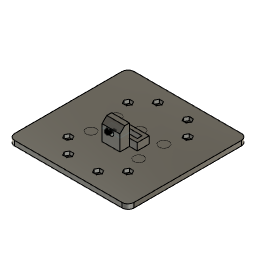
SidePanel-Back (Autodesk Fusion 360 design; units mm, degrees)
Autodesk Fusion 360 part; units mm, degrees
note: some values were not read from the file. Set by a fixed rule: which sketch regions a step uses.
sketch "Skizze1" plane through (0, 0, 0) normal (0, 0, 1) x (1, 0, 0)
  line L0 (0, 0) -> (100, 0)
  line L1 (100, 0) -> (100, 100)
  line L2 (100, 100) -> (0, 100)
  line L3 (0, 100) -> (0, 0)
  circle A0 centre (5, 95) radius 5
  circle A1 centre (5, 5) radius 5
  circle A2 centre (95, 5) radius 5
  circle A3 centre (95, 95) radius 5
  line L4 (39, 46.75) -> (61, 46.75)
  line L5 (61, 46.75) -> (61, 50.75)
  line L6 (61, 50.75) -> (39, 50.75)
  line L7 (39, 50.75) -> (39, 46.75)
  line L8 (39, 48.75) -> (61, 48.75)
  line L9 (50, 50.75) -> (50, 46.75)
  dimension "d1" = 100
  dimension "d2" = 100
  dimension "d5" = 22
  dimension "d6" = 4
  dimension "d7" = 50
  dimension "d8" = 48.75
  constraint horizontal L0
  constraint vertical L1
  constraint horizontal L2
  constraint vertical L3
  constraint coincident L0.start L3.end
  constraint tangent L2 A0
  constraint tangent L0 A1
  constraint tangent L1 A2
  constraint tangent L2 A3
  constraint horizontal L4
  constraint vertical L5
  constraint horizontal L6
  constraint vertical L7
  constraint midpoint L7 L8.start
  constraint midpoint L5 L8.end
  constraint midpoint L6 L9.start
  constraint midpoint L4 L9.end
  measures "d1" distance of L0.start L0.end
  measures "d2" distance of L0.start L2.end
  measures "d5" distance of L4.start L4.end
  measures "d6" distance of L4.start L6.end
  measures "d7" distance of L3 L9
  measures "d8" distance of L0 L8
extrude "Extrusion1" add sketch "Skizze1" along normal blind 4 contours L0 L1 L2 L3 A0 A1 A2 A3 | A1 | A2 | A0 | A3
sketch "Skizze2" plane through (0, 0, 4) normal (0, 0, 1) x (-1, 0, 0)
  line L0 (-39, -46.75) -> (-39, -50.75)
  line L1 (-39, -50.75) -> (-61, -50.75)
  line L2 (-61, -50.75) -> (-61, -46.75)
  line L3 (-61, -46.75) -> (-39, -46.75)
  arc A0 (-100, -95) -> (-95, -100) centre (-95, -95) ccw
  line L4 (-95, -100) -> (-5, -100)
  arc A1 (-5, -100) -> (0, -95) centre (-5, -95) ccw
  line L5 (0, -95) -> (0, -5)
  arc A2 (0, -5) -> (-5, 0) centre (-5, -5) ccw
  line L6 (-5, 0) -> (-95, 0)
  arc A3 (-95, 0) -> (-100, -5) centre (-95, -5) ccw
  line L7 (-100, -5) -> (-100, -95)
  line L8 (-39, -53.75) -> (-64, -53.75)
  line L9 (-64, -53.75) -> (-64, -43.75)
  line L10 (-64, -43.75) -> (-39, -43.75)
  line L11 (-39, -43.75) -> (-39, -53.75)
  line L12 (-39, -48.75) -> (-42, -48.75)
  arc A4 (-39, -53.75) -> (-39, -43.75) centre (-39, -48.75) ccw
  dimension "d9" = 3
  dimension "d10" = 3
  dimension "d11" = 3
  constraint horizontal L8
  constraint vertical L9
  constraint horizontal L10
  constraint vertical L11
  constraint collinear L0 L11
  constraint midpoint L11 L12.start
  constraint perpendicular L11 L12
  constraint coincident L12.start A4.centre
  measures "d9" distance of L1 L8
  measures "d10" distance of L3 L10
  measures "d11" distance of L2 L9
extrude "Extrusion2" add sketch "Skizze2" along normal blind 6 contours L0 L11 A4 | L1 L2 L3 L8 L9 L10 L11
sketch "Skizze3" plane through (0, 0, 0) normal (0, 0, -1) x (1, 0, 0)
  line L0 (39, -50.75) -> (39, -46.75)
  line L1 (39, -46.75) -> (61, -46.75)
  line L2 (61, -46.75) -> (61, -50.75)
  line L3 (61, -50.75) -> (39, -50.75)
  arc A0 (95, -100) -> (100, -95) centre (95, -95) ccw
  line L4 (100, -95) -> (100, -5)
  arc A1 (100, -5) -> (95, 0) centre (95, -5) ccw
  line L5 (95, 0) -> (5, 0)
  arc A2 (5, 0) -> (0, -5) centre (5, -5) ccw
  line L6 (0, -5) -> (0, -95)
  arc A3 (0, -95) -> (5, -100) centre (5, -95) ccw
  line L7 (5, -100) -> (95, -100)
  line L8 (23, -36) -> (3, -36)
  line L9 (3, -36) -> (3, -5)
  line L10 (3, -5) -> (23, -5)
  line L11 (23, -5) -> (23, -36)
  line L12 (23, -36) -> (18, -36)
  line L13 (18, -36) -> (18, -21)
  line L14 (18, -21) -> (23, -21)
  line L15 (23, -21) -> (23, -36)
  dimension "d15" = 20
  dimension "d16" = 31
  dimension "d17" = 5
  dimension "d18" = 3
  dimension "d62" = 5
  dimension "d63" = 15
  constraint horizontal L8
  constraint vertical L9
  constraint horizontal L10
  constraint vertical L11
  constraint horizontal L12
  constraint vertical L13
  constraint horizontal L14
  constraint vertical L15
  measures "d15" distance of L8.start L8.end
  measures "d16" distance of L8.start L10.end
  measures "d17" distance of L5 L10
  measures "d18" distance of L6 L9
  measures "d62" distance of L13.end L14.end
  measures "d63" distance of L12.end L13.end
extrude "Extrusion3" cut sketch "Skizze3" against normal blind 2 contours L8 L9 L10 L11 L13 L14
sketch "Skizze4" plane through (0, 0, 0) normal (0, 0, -1) x (1, 0, 0)
  line L0 (3, -36) -> (3, -5)
  line L1 (3, -5) -> (23, -5)
  line L2 (23, -5) -> (23, -21)
  line L3 (18, -36) -> (3, -36)
  line L4 (39, -50.75) -> (39, -46.75)
  line L5 (39, -46.75) -> (61, -46.75)
  line L6 (61, -46.75) -> (61, -50.75)
  line L7 (61, -50.75) -> (39, -50.75)
  arc A0 (95, -100) -> (100, -95) centre (95, -95) ccw
  line L8 (100, -95) -> (100, -5)
  arc A1 (100, -5) -> (95, 0) centre (95, -5) ccw
  line L9 (95, 0) -> (5, 0)
  arc A2 (5, 0) -> (0, -5) centre (5, -5) ccw
  line L10 (0, -5) -> (0, -95)
  arc A3 (0, -95) -> (5, -100) centre (5, -95) ccw
  line L11 (5, -100) -> (95, -100)
  line L12 (25, -25) -> (75, -25)
  line L13 (75, -25) -> (75, -75)
  line L14 (75, -75) -> (25, -75)
  line L15 (25, -75) -> (25, -25)
  circle A4 centre (25, -25) radius 1.75
  circle A5 centre (75, -25) radius 1.75
  circle A6 centre (75, -75) radius 1.75
  circle A7 centre (25, -75) radius 1.75
  line L16 (37.5, -12.5) -> (62.5, -12.5)
  line L17 (62.5, -12.5) -> (62.5, -87.5)
  line L18 (62.5, -87.5) -> (37.5, -87.5)
  line L19 (37.5, -87.5) -> (37.5, -12.5)
  circle A8 centre (37.5, -12.5) radius 1.75
  circle A9 centre (62.5, -12.5) radius 1.75
  circle A10 centre (62.5, -87.5) radius 1.75
  circle A11 centre (37.5, -87.5) radius 1.75
  line L20 (23, -21) -> (18, -21)
  line L21 (18, -21) -> (18, -36)
  dimension "d21" = 50
  dimension "d22" = 50
  dimension "d23" = 25
  dimension "d24" = 25
  dimension "d25" = 3.5
  dimension "d26" = 3.5
  dimension "d27" = 3.5
  dimension "d28" = 3.5
  dimension "d29" = 25
  dimension "d30" = 75
  dimension "d31" = 12.5
  dimension "d32" = 37.5
  dimension "d33" = 3.5
  dimension "d34" = 3.5
  dimension "d35" = 3.5
  dimension "d36" = 3.5
  constraint horizontal L12
  constraint vertical L13
  constraint horizontal L14
  constraint vertical L15
  constraint coincident L12.start L15.end
  constraint coincident L12.end L13.start
  constraint coincident L13.end L14.start
  constraint coincident L14.end L15.start
  constraint horizontal L16
  constraint vertical L17
  constraint horizontal L18
  constraint vertical L19
  constraint coincident L16.start L19.end
  constraint coincident L16.end L17.start
  constraint coincident L17.end L18.start
  constraint coincident L18.end L19.start
  measures "d21" distance of L12.start L12.end
  measures "d22" distance of L12.end L13.end
  measures "d23" distance of L8 L13
  measures "d24" distance of L11 L14
  measures "d25" diameter of A4
  measures "d26" diameter of A5
  measures "d27" diameter of A6
  measures "d28" diameter of A7
  measures "d29" distance of L16.start L16.end
  measures "d30" distance of L16.start L18.end
  measures "d31" distance of L9 L16
  measures "d32" distance of L8 L17
  measures "d33" diameter of A8
  measures "d34" diameter of A9
  measures "d35" diameter of A10
  measures "d36" diameter of A11
extrude "Extrusion4" cut sketch "Skizze4" against normal blind 4 contours L12 L15 A4 | L12 L15 A4 | L14 L15 A7 | L14 L15 A7 | L16 L19 A8 | L16 L19 A8 | L12 L13 A5 | L12 L13 A5 | L16 L17 A9 | L16 L17 A9 | L18 L19 A11 | L18 L19 A11 | L13 L14 A6 | L13 L14 A6 | L17 L18 A10 | L17 L18 A10
sketch "Skizze5" plane through (0, 0, 4) normal (0, 0, 1) x (-1, 0, 0)
  circle A0 centre (-37.5, -87.5) radius 1.75
  circle A1 centre (-25, -75) radius 1.75
  line L0 (-64, -53.75) -> (-64, -43.75)
  line L1 (-64, -43.75) -> (-39, -43.75)
  arc A2 (-39, -53.75) -> (-39, -43.75) centre (-39, -48.75) ccw
  line L2 (-39, -53.75) -> (-64, -53.75)
  arc A3 (-100, -95) -> (-95, -100) centre (-95, -95) ccw
  line L3 (-95, -100) -> (-5, -100)
  arc A4 (-5, -100) -> (0, -95) centre (-5, -95) ccw
  line L4 (0, -95) -> (0, -5)
  arc A5 (0, -5) -> (-5, 0) centre (-5, -5) ccw
  line L5 (-5, 0) -> (-95, 0)
  arc A6 (-95, 0) -> (-100, -5) centre (-95, -5) ccw
  line L6 (-100, -5) -> (-100, -95)
  line L7 (-34, -90.45) -> (-42, -90.45)
  line L8 (-34, -84.55) -> (-43, -84.55)
  line L9 (-20.1646, -77.9663) -> (-28.1646, -77.9393)
  line L10 (-20.1651, -72.05) -> (-29.1651, -72.05)
  line L11 (0, -50) -> (-100, -50)
  line L12 (-50, -100) -> (-50, 0)
  circle A7 centre (-50, -50) radius 3
  line L13 (-36.6952, -82.9939) -> (-32.6952, -89.9221)
  line L14 (-41.8048, -85.9439) -> (-37.3048, -93.7381)
  line L15 (-41.8048, -89.0561) -> (-37.8048, -82.1279)
  line L16 (-36.6952, -92.0061) -> (-32.1952, -84.2119)
  line L17 (-24.8488, -69.3292) -> (-20.8722, -76.2709)
  line L18 (-29.9722, -72.2879) -> (-25.4722, -80.0821)
  line L19 (-29.9866, -77.7044) -> (-25.9633, -70.7897)
  line L20 (-24.8627, -80.6621) -> (-20.3627, -72.8679)
  line L21 (-79.9722, -72.2879) -> (-75.4722, -80.0821)
  line L22 (-70.1646, -77.9663) -> (-78.1646, -77.9393)
  line L23 (-74.8627, -80.6621) -> (-70.3627, -72.8679)
  line L24 (-74.8488, -69.3292) -> (-70.8722, -76.2709)
  line L25 (-70.1651, -72.05) -> (-79.1651, -72.05)
  line L26 (-79.9866, -77.7044) -> (-75.9633, -70.7897)
  line L27 (-29.9722, -22.2879) -> (-25.4722, -30.0821)
  line L28 (-20.1646, -27.9663) -> (-28.1646, -27.9393)
  line L29 (-24.8627, -30.6621) -> (-20.3627, -22.8679)
  line L30 (-24.8488, -19.3292) -> (-20.8722, -26.2709)
  line L31 (-20.1651, -22.05) -> (-29.1651, -22.05)
  line L32 (-29.9866, -27.7044) -> (-25.9633, -20.7897)
  line L33 (-79.9722, -22.2879) -> (-75.4722, -30.0821)
  line L34 (-70.1646, -27.9663) -> (-78.1646, -27.9393)
  line L35 (-74.8627, -30.6621) -> (-70.3627, -22.8679)
  line L36 (-74.8488, -19.3292) -> (-70.8722, -26.2709)
  line L37 (-70.1651, -22.05) -> (-79.1651, -22.05)
  line L38 (-79.9866, -27.7044) -> (-75.9633, -20.7897)
  line L39 (-59, -84.55) -> (-68, -84.55)
  line L40 (-61.6952, -82.9939) -> (-57.6952, -89.9221)
  line L41 (-61.6952, -92.0061) -> (-57.1952, -84.2119)
  line L42 (-59, -90.45) -> (-67, -90.45)
  line L43 (-66.8048, -85.9439) -> (-62.3048, -93.7381)
  line L44 (-66.8048, -89.0561) -> (-62.8048, -82.1279)
  line L45 (-34, -9.55) -> (-43, -9.55)
  line L46 (-36.6952, -7.9939) -> (-32.6952, -14.9221)
  line L47 (-36.6952, -17.0061) -> (-32.1952, -9.2119)
  line L48 (-34, -15.45) -> (-42, -15.45)
  line L49 (-41.8048, -10.9439) -> (-37.3048, -18.7381)
  line L50 (-41.8048, -14.0561) -> (-37.8048, -7.1279)
  line L51 (-59, -9.55) -> (-68, -9.55)
  line L52 (-61.6952, -7.9939) -> (-57.6952, -14.9221)
  line L53 (-61.6952, -17.0061) -> (-57.1952, -9.2119)
  line L54 (-59, -15.45) -> (-67, -15.45)
  line L55 (-66.8048, -10.9439) -> (-62.3048, -18.7381)
  line L56 (-66.8048, -14.0561) -> (-62.8048, -7.1279)
  dimension "d40" = 2.95
  dimension "d41" = 2.95
  dimension "d42" = 2.95
  dimension "d43" = 2.95
  dimension "d78" = 360
  dimension "d80" = 360
  dimension "d83" = -50
  dimension "d84" = 50
  dimension "d87" = -25
  dimension "d88" = 75
  constraint parallel L3 L7
  constraint horizontal L8
  constraint horizontal L10
  constraint midpoint L4 L11.start
  constraint midpoint L6 L11.end
  constraint midpoint L3 L12.start
  constraint midpoint L5 L12.end
  constraint midpoint L11 A7.centre
  measures "d40" distance of A0.centre L7
  measures "d41" distance of A0.centre L8
  measures "d42" distance of A1.centre L9
  measures "d43" distance of A1.centre L10
extrude "Extrusion5" cut sketch "Skizze5" against normal blind 3 contours A0 | L7 L8 L13 L14 L15 L16 | L9 L10 L17 L18 L19 L20 | L21 L22 L23 L24 L25 L26 | L27 L28 L29 L30 L31 L32 | L33 L34 L35 L36 L37 L38 | L39 L40 L41 L42 L43 L44 | L45 L46 L47 L48 L49 L50 | L51 L52 L53 L54 L55 L56
sketch "Skizze6" plane through (0, 0, 4) normal (0, 0, 1) x (-1, 0, 0)
  line L0 (-26.6966, -72.05) -> (-23.2902, -72.05)
  line L1 (-23.3001, -77.9557) -> (-26.7065, -77.9443)
  line L2 (-39.2032, -84.55) -> (-35.7968, -84.55)
  line L3 (-35.7968, -90.45) -> (-39.2032, -90.45)
  line L4 (-64, -53.75) -> (-64, -43.75)
  line L5 (-64, -43.75) -> (-39, -43.75)
  arc A0 (-39, -53.75) -> (-39, -43.75) centre (-39, -48.75) ccw
  line L6 (-39, -53.75) -> (-64, -53.75)
  arc A1 (-100, -95) -> (-95, -100) centre (-95, -95) ccw
  line L7 (-95, -100) -> (-5, -100)
  arc A2 (-5, -100) -> (0, -95) centre (-5, -95) ccw
  line L8 (0, -95) -> (0, -5)
  arc A3 (0, -5) -> (-5, 0) centre (-5, -5) ccw
  line L9 (-5, 0) -> (-95, 0)
  arc A4 (-95, 0) -> (-100, -5) centre (-95, -5) ccw
  line L10 (-100, -5) -> (-100, -95)
  line L11 (-42.5, -43.75) -> (-57.5, -43.75)
  line L12 (-57.5, -43.75) -> (-57.5, -35.75)
  line L13 (-57.5, -35.75) -> (-42.5, -35.75)
  line L14 (-42.5, -35.75) -> (-42.5, -43.75)
  line L15 (-28.4097, -74.9943) -> (-26.6966, -72.05)
  line L16 (-23.2902, -72.05) -> (-21.5969, -75.0057)
  line L17 (-21.5969, -75.0057) -> (-23.3001, -77.9557)
  line L18 (-26.7065, -77.9443) -> (-28.4097, -74.9943)
  line L19 (-40.9064, -87.5) -> (-39.2032, -84.55)
  line L20 (-35.7968, -84.55) -> (-34.0936, -87.5)
  line L21 (-34.0936, -87.5) -> (-35.7968, -90.45)
  line L22 (-39.2032, -90.45) -> (-40.9064, -87.5)
  line L23 (-28.4097, -24.9943) -> (-26.6966, -22.05)
  line L24 (-26.6966, -22.05) -> (-23.2902, -22.05)
  line L25 (-23.2902, -22.05) -> (-21.5969, -25.0057)
  line L26 (-21.5969, -25.0057) -> (-23.3001, -27.9557)
  line L27 (-23.3001, -27.9557) -> (-26.7065, -27.9443)
  line L28 (-26.7065, -27.9443) -> (-28.4097, -24.9943)
  line L29 (-65.9064, -87.5) -> (-64.2032, -84.55)
  line L30 (-64.2032, -84.55) -> (-60.7968, -84.55)
  line L31 (-60.7968, -84.55) -> (-59.0936, -87.5)
  line L32 (-59.0936, -87.5) -> (-60.7968, -90.45)
  line L33 (-60.7968, -90.45) -> (-64.2032, -90.45)
  line L34 (-64.2032, -90.45) -> (-65.9064, -87.5)
  line L35 (-40.9064, -12.5) -> (-39.2032, -9.55)
  line L36 (-39.2032, -9.55) -> (-35.7968, -9.55)
  line L37 (-35.7968, -9.55) -> (-34.0936, -12.5)
  line L38 (-34.0936, -12.5) -> (-35.7968, -15.45)
  line L39 (-35.7968, -15.45) -> (-39.2032, -15.45)
  line L40 (-39.2032, -15.45) -> (-40.9064, -12.5)
  line L41 (-78.4097, -24.9943) -> (-76.6966, -22.05)
  line L42 (-76.6966, -22.05) -> (-73.2902, -22.05)
  line L43 (-73.2902, -22.05) -> (-71.5969, -25.0057)
  line L44 (-71.5969, -25.0057) -> (-73.3001, -27.9557)
  line L45 (-73.3001, -27.9557) -> (-76.7065, -27.9443)
  line L46 (-76.7065, -27.9443) -> (-78.4097, -24.9943)
  line L47 (-78.4097, -74.9943) -> (-76.6966, -72.05)
  line L48 (-76.6966, -72.05) -> (-73.2902, -72.05)
  line L49 (-73.2902, -72.05) -> (-71.5969, -75.0057)
  line L50 (-71.5969, -75.0057) -> (-73.3001, -77.9557)
  line L51 (-73.3001, -77.9557) -> (-76.7065, -77.9443)
  line L52 (-76.7065, -77.9443) -> (-78.4097, -74.9943)
  line L53 (-65.9064, -12.5) -> (-64.2032, -9.55)
  line L54 (-64.2032, -9.55) -> (-60.7968, -9.55)
  line L55 (-60.7968, -9.55) -> (-59.0936, -12.5)
  line L56 (-59.0936, -12.5) -> (-60.7968, -15.45)
  line L57 (-60.7968, -15.45) -> (-64.2032, -15.45)
  line L58 (-64.2032, -15.45) -> (-65.9064, -12.5)
  dimension "d64" = 15
  dimension "d65" = 42.5
  dimension "d66" = 8
  constraint horizontal L11
  constraint vertical L12
  constraint horizontal L13
  constraint vertical L14
  constraint coincident L5 L11.start
  measures "d64" distance of L12.end L13.end
  measures "d65" distance of L10 L12
  measures "d66" distance of L11.end L12.end
extrude "Extrusion6" add sketch "Skizze6" along normal blind 10 contours L5 L11 L12 L13 L14
sketch "Skizze8" plane through (0, 0, 14) normal (0, 0, 1) x (-1, 0, 0)
  line L0 (-42.5, -35.75) -> (-57.5, -35.75)
  line L1 (-57.5, -35.75) -> (-57.5, -43.75)
  line L2 (-57.5, -43.75) -> (-42.5, -43.75)
  line L3 (-42.5, -43.75) -> (-42.5, -35.75)
  line L4 (-50, -35.75) -> (-50, -39.75)
  line L5 (-50, -39.75) -> (-48.5, -39.75)
  line L6 (-48.5, -39.75) -> (-47.75, -35.75)
  dimension "d70" = 4
  dimension "d71" = 1.5
  dimension "d72" = 2.25
  constraint midpoint L0 L4.start
  constraint perpendicular L0 L4
  constraint perpendicular L4 L5
  constraint coincident L0 L6.end
  measures "d70" distance of L4.start L4.end
  measures "d71" distance of L4.end L5.end
  measures "d72" distance of L4.start L6.end
extrude "Extrusion7" add sketch "Skizze8" along normal blind 7
revolve "Drehen1" cut sketch "Skizze8" angle 360 about axis through (50, 35.75, 14) along (0, 1, 0) contours L0 L4 L5 L6
chamfer "Fase1" distance 4 angle 45 1 edges at (50, 35.75, 21)
sketch "Skizze9" plane through (0, 0, 0) normal (0, 0, -1) x (1, 0, 0)
  circle A0 centre (37.5, -87.5) radius 1.75
  circle A1 centre (62.5, -12.5) radius 1.75
  circle A2 centre (75, -25) radius 1.75
  circle A3 centre (25, -75) radius 1.75
  circle A4 centre (62.5, -87.5) radius 1.75
  circle A5 centre (37.5, -12.5) radius 1.75
  circle A6 centre (75, -75) radius 1.75
  circle A7 centre (25, -25) radius 1.75
  line L0 (23, -21) -> (18, -21)
  line L1 (18, -21) -> (18, -36)
  line L2 (18, -36) -> (3, -36)
  line L3 (3, -36) -> (3, -5)
  line L4 (3, -5) -> (23, -5)
  line L5 (23, -5) -> (23, -21)
  line L6 (39, -50.75) -> (39, -46.75)
  line L7 (39, -46.75) -> (61, -46.75)
  line L8 (61, -46.75) -> (61, -50.75)
  line L9 (61, -50.75) -> (39, -50.75)
  arc A8 (95, -100) -> (100, -95) centre (95, -95) ccw
  line L10 (100, -95) -> (100, -5)
  arc A9 (100, -5) -> (95, 0) centre (95, -5) ccw
  line L11 (95, 0) -> (5, 0)
  arc A10 (5, 0) -> (0, -5) centre (5, -5) ccw
  line L12 (0, -5) -> (0, -95)
  arc A11 (0, -95) -> (5, -100) centre (5, -95) ccw
  line L13 (5, -100) -> (95, -100)
  circle A12 centre (30, -39) radius 4.1
  circle A13 centre (70, -39) radius 4.1
  circle A14 centre (70, -60) radius 4.1
  circle A15 centre (30, -60) radius 4.1
  circle A16 centre (50, -60) radius 4.1
  dimension "d89" = 8.2
  dimension "d90" = 8.2
  dimension "d91" = 8.2
  dimension "d92" = 8.2
  dimension "d93" = 8.2
  dimension "d94" = 40
  dimension "d95" = 40
  dimension "d96" = 40
  dimension "d97" = 39
  dimension "d98" = 39
  dimension "d99" = 30
  dimension "d100" = 30
  dimension "d101" = 30
  dimension "d102" = 50
  dimension "d103" = 30
  measures "d89" diameter of A12
  measures "d90" diameter of A13
  measures "d91" diameter of A14
  measures "d92" diameter of A15
  measures "d93" diameter of A16
  measures "d94" distance of L13 A16.centre
  measures "d95" distance of L13 A15.centre
  measures "d96" distance of L13 A14.centre
  measures "d97" distance of L11 A13.centre
  measures "d98" distance of L11 A12.centre
  measures "d99" distance of L12 A12.centre
  measures "d100" distance of L10 A13.centre
  measures "d101" distance of L10 A14.centre
  measures "d102" distance of L10 A16.centre
  measures "d103" distance of L12 A15.centre
extrude "Extrusion8" cut sketch "Skizze9" against normal blind 3.5 contours A12 | A13 | A14 | A15 | A16
equation "d8 = 50 mm - 1.25 mm"
equation "d65 = ( ( 100 - 15 ) / 2 ) * 1 mm"
